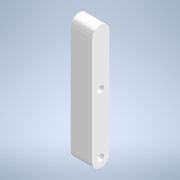
# Autodesk Inventor part: ServoArm
Saved by Autodesk Inventor 2021 (Build 250183000, 183)
## iProperties
Created: 2021-05-22
Part Number: ServoArm
Material: PC/ABS Plastic
Document SubType Name: Modeling
Designer: sami8
Density: 0.357273 g/cm^3
Appearance: Smooth - White
Author: sami8
Autodesk Inventor part; units mm, degrees
ref_plane "YZ Plane" through (0, 0, 0) normal (1, 0, 0) x (0, 1, 0)
ref_plane "XZ Plane" through (0, 0, 0) normal (0, 1, 0) x (-1, 0, 0)
ref_plane "XY Plane" through (0, 0, 0) normal (0, 0, 1) x (1, 0, 0)
sketch "Sketch1" plane through (0, 0, 0) normal (1, 0, 0) x (0, 1, 0)
  line L0 (0, 0) -> (50, 0) construction
  line L1 (0, -4) -> (50, -4)
  line L2 (50, 4) -> (0, 4)
  arc A0 (0, 4) -> (0, -4) centre (0, 0) ccw
  arc A1 (50, -4) -> (50, 4) centre (50, 0) ccw
  circle A2 centre (0, 0) radius 1.55
  circle A3 centre (8, 0) radius 1.55
  point P0 (25, 0)
  dimension "d0" = 50
  dimension "d1" = 8
  dimension "d2" = 3.1
  dimension "d3" = 3.1
  dimension "d4" = 8
  constraints: 8 end point, 4 centre point, 4 point on circle, 4 tangent, 1 coincident, 1 horizontal, 1 midpoint, 1 parallel, 1 point on line
  measures "d0" distance of L0.start L0.end
  measures "d1" diameter of A1
  measures "d2" diameter of A2
  measures "d3" diameter of A3
  measures "d4" distance of A2.centre A3.centre
extrude "Extrusion1" add sketch "Sketch1" along normal blind 7
body "Solid1"
